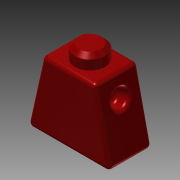
# Autodesk Inventor part: Lego Body
Saved by Autodesk Inventor 2013 (Build 170138000, 138)
## iProperties
Created: 2013-09-06
Part Number: Lego Body
Material: Generic
Document SubType Name: Modeling
Designer: 200395375
Density: 1 g/cm^3
Author: 200395375
Autodesk Inventor part; units mm, degrees
ref_plane "YZ Plane" through (0, 0, 0) normal (1, 0, 0) x (0, 1, 0)
ref_plane "XZ Plane" through (0, 0, 0) normal (0, 1, 0) x (-1, 0, 0)
ref_plane "XY Plane" through (0, 0, 0) normal (0, 0, 1) x (1, 0, 0)
sketch "Sketch1" plane through (0, 0, 0) normal (0, 1, 0) x (-1, 0, 0)
  line L0 (0, 0) -> (15.44, 0)
  line L1 (2.85, 12.77) -> (12.59, 12.77)
  line L2 (12.59, 12.77) -> (15.44, 0)
  line L3 (2.85, 12.77) -> (0, 0)
  dimension "d0" = 15.44
  dimension "d1" = 9.74
  dimension "d2" = 12.77
  constraints: 8 end point, 1 horizontal, 1 parallel
  measures "d0" distance of L0.start L0.end
  measures "d1" distance of L1.start L1.end
  measures "d2" vertical distance of L1.start L0.start
extrude "Body" add sketch "Sketch1" along normal blind 8
fillet "Edge" radius 0.75 12 edges at (-12.59, 4, 12.77) (-2.85, 4, 12.77) (0, 4, 0) (-15.44, 4, 0) (-7.72, 0, 0) (-7.72, 8, 0) (-14.015, 0, 6.385) (-7.72, 0, 12.77) (-1.425, 0, 6.385) (-1.425, 8, 6.385) (-7.72, 8, 12.77) (-14.015, 8, 6.385)
sketch "Sketch5" plane through (-11.9889, 0.75, 12.77) normal (0, 0, 1) x (1, 0, 0)
  circle A0 centre (4.2689, 3.25) radius 2.81
  point P0 (11.9889, -0.75)
  dimension "d9" = 5.62
  constraints: 1 centre point
  measures "d9" diameter of A0
extrude "Head Joint" add sketch "Sketch5" along normal blind 2.5
chamfer "Head Edge" distance 0.75 angle 45 1 edges at (-10.53, 4, 15.27)
sketch "Sketch6" plane through (-0.9358, 0.75, 0) normal (0, 0, -1) x (-1, 0, 0)
  line L0 (13.5683, 6.5) -> (13.5683, 0) projected
  line L1 (0, 0) -> (0, 6.5) projected
  circle A0 centre (3.25, 3.25) radius 1.5
  circle A1 centre (10.3183, 3.25) radius 1.5
  point P0 (-0.9358, -0.75)
  dimension "d15" = 3
  dimension "d16" = 3
  dimension "d17" = 3.25
  dimension "d18" = 3.25
  constraints: 2 centre point
  measures "d15" diameter of A0
  measures "d16" diameter of A1
  measures "d17" distance from line of L0 A1.centre
  measures "d18" distance from line of L1 A0.centre
extrude "Leg Joint" cut sketch "Sketch6" against normal blind 2.5
chamfer "Leg Edge" distance 0.75 angle 45 4 edges at (-2.6858, 4, 0) (-9.7542, 4, 0) (-9.7542, 4, 2.5) (-2.6858, 4, 2.5)
sketch "Sketch7" plane through (-0.2038, 0.75, 0.9134) normal (0.976, 0, 0.2178) x (0.2178, 0, -0.976)
  line L0 (-11.5473, 0) -> (-11.5473, 6.5) projected
  circle A0 centre (-8.2973, 3.25) radius 1.5
  point P0 (0.9358, -0.75)
  dimension "d24" = 3
  dimension "d25" = 3.25
  constraints: 1 centre point
  measures "d24" diameter of A0
  measures "d25" distance from line of L0 A0.centre
extrude "Arm Joint1" cut sketch "Sketch7" against normal blind 2.5
fillet "Arm Edge1" radius 0.75 2 edges at (-4.7798, 4, 9.9304) (-2.3379, 4, 10.4754)
sketch "Sketch8" plane through (-12.7209, 0.75, 12.1834) normal (-0.976, 0, 0.2178) x (0.2178, 0, 0.976)
  line L0 (0, 6.5) -> (0, 0) projected
  circle A0 centre (-3.25, 3.25) radius 1.5
  point P0 (-9.12, -0.75)
  dimension "d29" = 3
  dimension "d30" = 3.25
  constraints: 1 centre point
  measures "d29" diameter of A0
  measures "d30" distance from line of L0 A0.centre
extrude "Arm Joint2" cut sketch "Sketch8" against normal blind 2.5
fillet "Arm Edge2" radius 0.75 2 edges at (-13.7556, 4, 7.5474) (-11.3136, 4, 7.0024)
body "Solid1"
